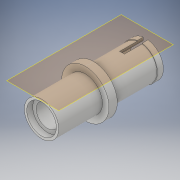
# Autodesk Inventor part: axle
Saved by Autodesk Inventor 2018 (Build 220112000, 112)
## iProperties
Created: 2019-01-10
Part Number: axle
Material: Generic
Document SubType Name: Modeling
Designer: mimss21
Density: 1 g/cm^3
Appearance: Default
Author: mimss21
Autodesk Inventor part; units mm, degrees
ref_plane "YZ Plane" through (0, 0, 0) normal (1, 0, 0) x (0, 1, 0)
ref_plane "XY Plane" through (0, 0, 0) normal (0, 0, 1) x (1, 0, 0)
sketch "Sketch1" plane through (0, 0, 0) normal (0, 0, 1) x (1, 0, 0)
  circle A0 centre (0, 0) radius 5.08
  dimension "d0" = 10.16
  constraints: 1 centre point, 1 coincident
  measures "d0" diameter of A0
extrude "Extrusion1" add sketch "Sketch1" along normal blind 12.954
sketch "Sketch2" plane through (0, 0, 12.954) normal (0, 0, 1) x (1, 0, 0)
  circle A0 centre (0, 0) radius 3.683
  dimension "d3" = 7.366
  constraints: 1 centre point, 1 coincident
  measures "d3" diameter of A0
extrude "Extrusion2" add sketch "Sketch2" along normal blind 9.398
sketch "Sketch4" plane through (0, 0, 22.352) normal (0, 0, 1) x (1, 0, 0)
  circle A0 centre (0, 0) radius 2.413
  dimension "d9" = 4.826
  constraints: 1 centre point, 1 coincident
  measures "d9" diameter of A0
extrude "Extrusion3" cut sketch "Sketch4" against normal blind 9.652
sketch "Sketch5" plane through (0, 0, 22.352) normal (0, 0, 1) x (1, 0, 0)
  circle A0 centre (0, 0) radius 3.175
  dimension "d12" = 6.35
  constraints: 1 centre point, 1 coincident
  measures "d12" diameter of A0
extrude "Extrusion4" cut sketch "Sketch5" against normal blind 1.27
sketch "Sketch6" plane through (0, 0, 0) normal (0, 0, -1) x (-1, 0, 0)
  circle A0 centre (0, 0) radius 2.413
  dimension "d15" = 4.826
  constraints: 1 centre point, 1 coincident
  measures "d15" diameter of A0
extrude "Extrusion5" cut sketch "Sketch6" against normal blind 11.176
sketch "Sketch7" plane through (0, 0, 0) normal (0, 0, -1) x (-1, 0, 0)
  circle A0 centre (0, 0) radius 3.175
  dimension "d18" = 6.35
  constraints: 1 centre point, 1 coincident
  measures "d18" diameter of A0
extrude "Extrusion6" cut sketch "Sketch7" against normal blind 6.35
sketch "Sketch8" plane through (0, 0, 0) normal (0, 0, -1) x (-1, 0, 0)
  circle A0 centre (0, 0) radius 3.683
  circle A1 centre (0, 0) radius 5.2614
  dimension "d21" = 7.366
  constraints: 2 centre point, 2 coincident
  measures "d21" diameter of A0
extrude "Extrusion7" cut sketch "Sketch8" against normal blind 11.176
sketch "Sketch9" plane through (0, 0, 0) normal (0, 0, -1) x (-1, 0, 0)
  circle A0 centre (0, 0) radius 3.81
  dimension "d24" = 7.62
  constraints: 1 centre point, 1 coincident
  measures "d24" diameter of A0
extrude "Extrusion8" add sketch "Sketch9" against normal blind 1.27
sketch "Sketch10" plane through (0, 0, 0) normal (0, 0, -1) x (-1, 0, 0)
  circle A0 centre (0, 0) radius 3.175
  constraints: 1 centre point, 1 coincident
extrude "Extrusion9" cut sketch "Sketch10" against normal blind 1.27
ref_plane "Work Plane1" through (0, 5.08, 0) normal (0, 1, 0) x (-1, 0, 0)
sketch "Sketch13" plane through (0, 5.08, 0) normal (0, 1, 0) x (-1, 0, 0)
  line L0 (0, 0) -> (-0.508, 0)
  line L1 (-0.508, 0) -> (-0.508, 5.08)
  line L2 (-0.508, 5.08) -> (0, 5.08)
  line L3 (0, 5.08) -> (0, 0)
  line L4 (0, 0) -> (0.508, 0)
  line L5 (0.508, 0) -> (0.508, 5.08)
  line L6 (0.508, 5.08) -> (0, 5.08)
  line L7 (0, 5.08) -> (0, 0)
  dimension "d30" = 5.08
  dimension "d31" = 0.508
  dimension "d32" = 0.508
  dimension "d33" = 5.08
  constraints: 16 end point, 4 parallel, 2 horizontal, 2 perpendicular
  measures "d30" distance of L0.end L1.end
  measures "d31" distance of L1.end L2.end
  measures "d32" distance of L5.end L6.end
  measures "d33" distance of L4.end L5.end
extrude "Extrusion10" cut sketch "Sketch13" against normal blind 10.16
body "Solid1"
